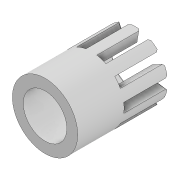
# Autodesk Inventor part: Axis 5 Drive Rod
Saved by Autodesk Inventor 2020 (Build 240168000, 168)
## iProperties
Created: 2021-06-29
Part Number: Axis 5 Drive Rod
Material: Generic
Document SubType Name: Modeling
Designer: Coy
Density: 1 g/cm^3
Appearance: Default
Author: Coy
Autodesk Inventor part; units mm, degrees
ref_plane "YZ Plane" through (0, 0, 0) normal (1, 0, 0) x (0, 1, 0)
ref_plane "XZ Plane" through (0, 0, 0) normal (0, 1, 0) x (-1, 0, 0)
ref_plane "XY Plane" through (0, 0, 0) normal (0, 0, 1) x (1, 0, 0)
sketch "Sketch1" plane through (0, 0, 0) normal (0, 0, 1) x (1, 0, 0)
  circle A0 centre (0, 0) radius 6
  circle A1 centre (0, 0) radius 4
  dimension "d0" = 12
  dimension "d1" = 8
  constraints: 2 centre point, 2 coincident
  measures "d0" diameter of A0
  measures "d1" diameter of A1
extrude "Extrusion1" add sketch "Sketch1" along normal blind 8.5
sketch "Sketch2" plane through (0, 0, 0) normal (0, 0, -1) x (-1, 0, 0)
  circle A0 centre (0, 0) radius 6 projected
  circle A1 centre (0, 0) radius 4 projected
  circle A2 centre (0, 0) radius 4 projected
  line L0 (-0.6667, 3.9441) -> (-1, 5.9161)
  circle A3 centre (0, 0) radius 6 projected
  line L1 (0.6667, 3.9441) -> (1, 5.9161)
  line L2 (0, 0) -> (0, 11.4601) construction
  line L3 (-2.8576, 2.7989) -> (-4.2864, 4.1984)
  line L4 (-1.7789, 3.5827) -> (-2.6684, 5.374)
  line L5 (-3.957, 0.5847) -> (-5.9355, 0.8771)
  line L6 (-3.545, 1.8528) -> (-5.3175, 2.7792)
  line L7 (-3.545, -1.8528) -> (-5.3175, -2.7792)
  line L8 (-3.957, -0.5847) -> (-5.9355, -0.8771)
  line L9 (-1.7789, -3.5827) -> (-2.6684, -5.374)
  line L10 (-2.8576, -2.7989) -> (-4.2864, -4.1984)
  line L11 (0.6667, -3.9441) -> (1, -5.9161)
  line L12 (-0.6667, -3.9441) -> (-1, -5.9161)
  line L13 (2.8576, -2.7989) -> (4.2864, -4.1984)
  line L14 (1.7789, -3.5827) -> (2.6684, -5.374)
  line L15 (3.957, -0.5847) -> (5.9355, -0.8771)
  line L16 (3.545, -1.8528) -> (5.3175, -2.7792)
  line L17 (3.545, 1.8528) -> (5.3175, 2.7792)
  line L18 (3.957, 0.5847) -> (5.9355, 0.8771)
  line L19 (1.7789, 3.5827) -> (2.6684, 5.374)
  line L20 (2.8576, 2.7989) -> (4.2864, 4.1984)
  dimension "d4" = 2
  dimension "d5" = 1
  dimension "d8" = 360
  constraints: 42 end point, 1 vertical, 71 other
  measures "d4" distance of L1.end L0.end
  measures "d5" distance from line of L2 L0.end
extrude "Extrusion2" add sketch "Sketch2" along normal blind 8 contours L18 A1 L17 A0 | A0 L16 A1 L15 | L20 A1 L19 A0 | A0 L14 A1 L13 | L1 A1 L0 A0 | A0 L12 A1 L11 | L4 A1 L3 A0 | A0 L10 A1 L9 | L6 A1 L5 A0 | A0 L8 A1 L7
chamfer "Chamfer1" distance 0.3 angle 45 30 edges at (3.572, 3.4987, -8) (2.2236, 4.4783, -8) (0.8333, 4.9301, -8) (-0.8333, 4.9301, -8) (-2.2236, 4.4783, -8) (-3.572, 3.4987, -8) (-4.4313, 2.316, -8) (-4.9463, 0.7309, -8) (-4.9463, -0.7309, -8) (-4.4313, -2.316, -8) (-3.572, -3.4987, -8) (-2.2236, -4.4783, -8) (-0.8333, -4.9301, -8) (0.8333, -4.9301, -8) (2.2236, -4.4783, -8) (3.572, -3.4987, -8) (4.4313, -2.316, -8) (4.9463, -0.7309, -8) (4.9463, 0.7309, -8) (4.4313, 2.316, -8) (-2.3511, 3.2361, -8) (-3.8042, 1.2361, -8) (-3.8042, -1.2361, -8) (-2.3511, -3.2361, -8) (0, -4, -8) (2.3511, -3.2361, -8) (3.8042, -1.2361, -8) (3.8042, 1.2361, -8) (2.3511, 3.2361, -8) (0, 4, -8)
body "Solid1"
